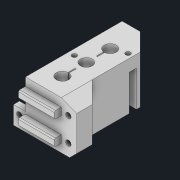
# Autodesk Inventor part: z-bottom
Saved by Autodesk Inventor 2021 (Build 250183000, 183)
## iProperties
Created: 2021-03-14
Part Number: z-bottom
Material: Generic
Document SubType Name: Modeling
Designer: Alex
Density: 1 g/cm^3
Appearance: Default
Author: Alex
## iProperties of the stored document _3DPrint.ipt
Created: 2021-05-20
Part Number: _3DPrint
Material: Generic
Document SubType Name: Modeling
Designer: arbra
Density: 1 g/cm^3
Appearance: Default
Author: arbra
Autodesk Inventor part; units mm, degrees
ref_plane "YZ Plane" through (0, 0, 0) normal (1, 0, 0) x (0, 1, 0)
ref_plane "XZ Plane" through (0, 0, 0) normal (0, 1, 0) x (-1, 0, 0)
sketch "Sketch1" plane through (0, 0, 0) normal (0, 1, 0) x (-1, 0, 0)
  circle A0 centre (0, 0) radius 5
  line L0 (-23.6, 0) -> (36.6, 0) construction
  line L1 (0, -52.2) -> (0, 61.2) construction
  circle A1 centre (0, 20) radius 5.125
  circle A2 centre (0, -20) radius 5.125
  circle A3 centre (-10, 0) radius 2
  circle A4 centre (11, 24) radius 2
  line L2 (0, 45) -> (15, 30)
  line L3 (15, 30) -> (15, -10)
  line L4 (15, -10) -> (28, -23)
  line L5 (28, -23) -> (28, -36)
  line L6 (28, -36) -> (-15, -36)
  line L7 (-15, -36) -> (-15, 45)
  line L8 (-15, 45) -> (0, 45)
  line L9 (0.375, 14.8887) -> (0.375, 8.8887)
  line L10 (0.375, 8.8887) -> (-0.375, 8.8887)
  line L11 (-0.375, 8.8887) -> (-0.375, 14.8887)
  line L12 (0.375, -14.8887) -> (0.375, -8.8887)
  line L13 (0.375, -8.8887) -> (-0.375, -8.8887)
  line L14 (-0.375, -8.8887) -> (-0.375, -14.8887)
  dimension "d0" = 10
  dimension "d1" = 10.25
  dimension "d3" = 40
  dimension "d4" = 4
  dimension "d5" = 11
  dimension "d6" = 4
  dimension "d9" = 10
  dimension "d10" = 4
  dimension "d13" = 45
  dimension "d14" = 15
  dimension "d16" = 16
  dimension "d17" = 13
  dimension "d18" = 45
  dimension "d19" = 25
  dimension "d24" = 0.75
  dimension "d25" = 6
  dimension "d106" = 13
  constraints: 26 end point, 5 centre point, 5 perpendicular, 5 symmetric about line, 4 point on line, 2 equal radius, 2 point on circle, 2 vertical, 1 coincident, 1 parallel, 1 other
  measures "d0" diameter of A0
  measures "d1" diameter of A1
  measures "d3" distance of A2.centre A1.centre
  measures "d4" diameter of A4
  measures "d5" horizontal distance of A4.centre A1.centre
  measures "d6" vertical distance of A4.centre A1.centre
  measures "d9" distance of A3.centre A0.centre
  measures "d10" distance from line of L3 A4.centre
  measures "d13" angle of L3 L4
  measures "d14" distance from line of L7 A0.centre
  measures "d16" distance from line of L6 A2.centre
  measures "d17" distance of L4.end L5.end
  measures "d18" angle of L2 L8
  measures "d19" distance from line of L8 A1.centre
  measures "d24" distance of L9.end L10.end
  measures "d25" distance of L9.start L9.end
  measures "d106" distance between parallel lines of L5 L3
extrude "Extrusion1" add sketch "Sketch1" along normal blind 40
sketch "Sketch2" plane through (0, 0, 0) normal (0, -1, 0) x (1, 0, 0)
  circle A0 centre (0, 0) radius 5 projected
extrude "Extrusion2" add sketch "Sketch2" against normal blind 20
sketch "Sketch3" plane through (0, 0, 0) normal (0, -1, 0) x (1, 0, 0)
  arc A0 (-0.375, -14.8887) -> (0.375, -14.8887) centre (0, -20) ccw projected
  circle A1 centre (0, -20) radius 2.5
  line L0 (-36.6, 0) -> (23.6, 0) construction
  line L1 (0.375, -14.8887) -> (0.375, -8.8887) projected
  line L2 (-0.375, -8.8887) -> (-0.375, -14.8887) projected
  line L3 (0.375, -8.8887) -> (-0.375, -8.8887) projected
  line L4 (-0.375, -14.8887) -> (-0.375, -17.5283)
  line L5 (0.375, -14.8887) -> (0.375, -17.5283)
  line L6 (-0.375, -22.4717) -> (-0.375, -24.9717)
  line L7 (-0.375, -24.9717) -> (0.375, -24.9717)
  line L8 (0.375, -24.9717) -> (0.375, -22.4717)
  arc A2 (0.375, 14.8887) -> (-0.375, 14.8887) centre (0, 20) ccw projected
  line L9 (-0.375, 14.8887) -> (-0.375, 8.8887) projected
  line L10 (0.375, 8.8887) -> (0.375, 14.8887) projected
  line L11 (-0.375, 8.8887) -> (0.375, 8.8887) projected
  circle A3 centre (0, 20) radius 2.5
  line L12 (-0.375, 14.8887) -> (-0.375, 17.5283)
  line L13 (0.375, 14.8887) -> (0.375, 17.5283)
  line L14 (-0.375, 22.4717) -> (-0.375, 24.9717)
  line L15 (-0.375, 24.9717) -> (0.375, 24.9717)
  line L16 (0.375, 24.9717) -> (0.375, 22.4717)
  line L17 (-0.375, -8.8887) -> (-0.375, -14.8887) projected
  arc A4 (0.375, -14.8887) -> (-0.375, -14.8887) centre (0, -20) ccw
  arc A5 (-0.375, 14.8887) -> (0.375, 14.8887) centre (0, 20) ccw
  point P0 (0, 0)
  dimension "d26" = 5
  dimension "d27" = 2.5
  dimension "d30" = 5.125
  dimension "d31" = 5.125
  constraints: 20 end point, 12 point on circle, 8 symmetric about line, 4 centre point, 3 vertical, 2 collinear, 1 coincident, 1 horizontal, 1 perpendicular, 2 other
  measures "d26" diameter of A1
  measures "d27" distance of L6.start L6.end
  measures "d30" radius of A4
  measures "d31" radius of A0
extrude "Extrusion3" add sketch "Sketch3" against normal blind 3.5 contours L4 A1 L6 L7 L8 L5 A0 | L2 L3 L1 A4 | L13 A3 L16 L15 L14 L12 A2 | L10 L11 L9 A5
sketch "Sketch4" plane through (15, 0, 45) normal (1, 0, 0) x (0, 0, -1)
  line L0 (81, 0) -> (81, 40) construction
  line L1 (81, 33.145) -> (85.85, 33.145)
  line L2 (86.85, 32.145) -> (86.85, 27.855)
  line L3 (85.85, 26.855) -> (81, 26.855)
  line L4 (81, 26.855) -> (81, 33.145)
  line L5 (81, 20) -> (108.6331, 20) construction
  line L6 (0, 40) -> (81, 40) construction
  line L7 (85.85, 33.145) -> (86.85, 32.145)
  line L8 (85.85, 26.855) -> (86.85, 27.855)
  line L9 (81, 6.855) -> (85.85, 6.855)
  line L10 (86.85, 7.855) -> (86.85, 12.145)
  line L11 (85.85, 13.145) -> (81, 13.145)
  line L12 (81, 13.145) -> (81, 6.855)
  line L13 (85.85, 6.855) -> (86.85, 7.855)
  line L14 (85.85, 13.145) -> (86.85, 12.145)
  point P0 (45, 0)
  point P1 (86.85, 26.855)
  point P2 (86.85, 33.145)
  point P3 (86.85, 13.145)
  point P4 (86.85, 6.855)
  dimension "d32" = 6.855
  dimension "d33" = 5.85
  dimension "d34" = 6.29
  dimension "d35" = 1
  dimension "d36" = 1
  dimension "d37" = 1
  dimension "d38" = 1
  constraints: 26 end point, 9 point on line, 8 symmetric about line, 2 horizontal, 2 parallel, 1 midpoint, 1 perpendicular
  measures "d32" distance between parallel lines of L1 L6
  measures "d33" distance of L1.start point (86.85, 33.145)
  measures "d34" distance between parallel lines of L3 L1
  measures "d35" distance of L1.end point (86.85, 33.145)
  measures "d36" distance of L2.start point (86.85, 33.145)
  measures "d37" distance of L3.start point (86.85, 26.855)
  measures "d38" distance of L2.end point (86.85, 26.855)
extrude "Extrusion4" add sketch "Sketch4" against normal up to surface (43 mm away)
sketch "Sketch5" plane through (15, 27.855, -41.85) normal (0, 0, -1) x (-1, 0, 0)
  line L0 (30, -27.855) -> (30, 12.145) construction
  line L1 (0, 5.29) -> (43, 5.29) projected
  line L2 (36, 5.29) -> (36, -1) construction
  line L3 (43, -1) -> (0, -1) projected
  circle A0 centre (36, 2.145) radius 2.25
  line L4 (0, -27.855) -> (0, 12.145) projected
  line L5 (0, -7.855) -> (43, -7.855) construction
  line L6 (43, -27.855) -> (43, 12.145) projected
  circle A1 centre (36, -17.855) radius 2.25
  point P0 (15, -27.855)
  dimension "d41" = 4.5
  dimension "d42" = 6
  constraints: 4 end point, 3 midpoint, 2 centre point, 2 point on line, 1 symmetric about line, 1 vertical, 1 other
  measures "d41" diameter of A0
  measures "d42" distance from line of L0 A0.centre
extrude "Extrusion5" cut sketch "Sketch5" against normal through all contours A0 | A1
ref_plane "Work Plane1" through (-15, 0, -10) normal (0, 0, 1) x (0, 1, 0)
sketch "Sketch6" plane through (-15, 0, -10) normal (0, 0, 1) x (0, 1, 0)
  circle A0 centre (30, 6) radius 2.25 projected
  circle A1 centre (30, 6) radius 3.75
  circle A2 centre (10, 6) radius 2.25 projected
  circle A3 centre (10, 6) radius 3.75
  point P0 (0, -15)
  dimension "d46" = 7.5
  dimension "d47" = 7.5
  constraints: 2 centre point, 2 coincident
  measures "d46" diameter of A1
  measures "d47" diameter of A3
extrude "Extrusion6" cut sketch "Sketch6" against normal blind 21 contours A0 | A1 | A2 | A3
sketch "Sketch7" plane through (15, 27.855, -41.85) normal (0, 0, -1) x (-1, 0, 0)
  line L0 (0, -27.855) -> (0, 12.145) projected
  line L1 (0, -7.855) -> (43, -7.855) construction
  line L2 (43, -27.855) -> (43, 12.145) projected
  line L3 (0, -15.71) -> (0, -20)
  line L4 (0, -12.855) -> (-10, -12.855)
  line L5 (-10, -12.855) -> (-10, -27.855)
  line L6 (-10, -27.855) -> (0, -27.855)
  line L7 (0, -27.855) -> (0, -12.855)
  line L8 (15, -27.855) -> (0, -27.855) projected
  point P0 (0, 0)
  point P1 (0, 4.29)
  point P2 (0, -17.855)
  point P3 (0, -12.855)
  point P4 (-10, -20.355)
  dimension "d63" = 10
  dimension "d64" = 5
  constraints: 12 end point, 3 midpoint, 2 collinear, 2 symmetric about line, 1 horizontal, 1 vertical
  measures "d63" distance of L4.start L5.start
  measures "d64" distance between parallel lines of L4 L1
extrude "Extrusion7" add sketch "Sketch7" against normal up to surface (86.85 mm away)
sketch "Sketch9" plane through (-28, 27.855, -41.85) normal (0, 0, -1) x (-1, 0, 0)
  arc A0 (-6.3207, 0) -> (-6.3207, 4.29) centre (-7, 2.145) ccw projected
  line L0 (-43, -6.9275) -> (0, -7.855) construction
  line L1 (0, -14.71) -> (0, -1) projected
  circle A1 centre (-48, -17.855) radius 2.25
  line L2 (-43, -12.855) -> (-53, -12.855) projected
  arc A2 (-7.6793, -15.71) -> (-7.6793, -20) centre (-7, -17.855) ccw projected
  line L3 (-7, -17.855) -> (-48, -17.855) construction
  line L4 (-48, -12.855) -> (-48, -17.855) construction
  point P0 (-28, -27.855)
  constraints: 6 end point, 2 midpoint, 1 centre point, 1 equal radius, 1 horizontal, 1 vertical
extrude "Extrusion9" cut sketch "Sketch9" against normal through all
sketch "Sketch10" plane through (0, 0, 45) normal (0, 0, 1) x (1, 0, 0)
  circle A0 centre (20, 10) radius 2.25 projected
  circle A1 centre (20, 10) radius 3.5
  point P0 (0, 0)
  dimension "d59" = 7
  constraints: 1 centre point, 1 coincident
  measures "d59" diameter of A1
extrude "Extrusion10" cut sketch "Sketch10" against normal blind 70 contours A0 | A1
sketch "Sketch11" plane through (25, 0, -41.85) normal (1, 0, 0) x (0, 0, -1)
  line L0 (-1, 13.145) -> (-5.85, 13.145) projected
  line L1 (-5.85, 13.145) -> (-5.85, 15) projected
  line L2 (0, 15) -> (-5.85, 15) projected
  line L3 (0, 12.145) -> (0, 15) projected
  line L4 (0, 12.145) -> (-1, 13.145) projected
  line L5 (-5.85, 13.145) -> (-5.85, 6.855) projected
  line L6 (0, 0) -> (0, 7.855) projected
  line L7 (-1, 6.855) -> (0, 7.855) projected
  line L8 (-5.85, 6.855) -> (-1, 6.855) projected
  line L9 (-5.85, 0) -> (-5.85, 6.855) projected
  line L10 (-5.85, 6.855) -> (-5.85, 0)
  line L11 (0, 0) -> (-86.85, 0) projected
  line L12 (-5.85, 0) -> (0, 0)
  point P0 (-41.85, 0)
  constraints: 4 end point, 1 collinear, 1 vertical
extrude "Extrusion11" cut sketch "Sketch11" against normal through all
sketch "Sketch12" plane through (15, 27.855, -41.85) normal (1, 0, 0) x (0, 0, -1)
  line L0 (-43.85, 12.145) -> (-39.85, 12.145) projected
  line L1 (-44.85, -27.855) -> (-38.85, -27.855)
  line L2 (-38.85, -27.855) -> (-38.85, 2.145)
  line L3 (-38.85, 2.145) -> (-44.85, 2.145)
  line L4 (-44.85, 2.145) -> (-44.85, -27.855)
  line L5 (-41.85, 12.145) -> (-41.85, 2.145)
  line L6 (-31.85, -27.855) -> (-71.85, -27.855) projected
  point P0 (-41.85, -27.855)
  dimension "d72" = 10
  dimension "d74" = 6
  constraints: 10 end point, 2 midpoint, 2 parallel, 2 perpendicular, 1 collinear, 1 horizontal, 1 other
  measures "d72" distance between parallel lines of L3 L0
  measures "d74" distance of L1.start L1.end
extrude "Extrusion12" cut sketch "Sketch12" against normal blind 8
sketch "Sketch13" plane through (-15, 10, -10) normal (-1, 0, 0) x (0, 0, 1)
  line L0 (32, 30) -> (36, 30) projected
  line L1 (34, 30) -> (34, 20)
  line L2 (31, -10) -> (37, -10)
  line L3 (37, -10) -> (37, 20)
  line L4 (37, 20) -> (31, 20)
  line L5 (31, 20) -> (31, -10)
  line L6 (0, -10) -> (40, -10) projected
  dimension "d79" = 6
  dimension "d110" = 10
  constraints: 10 end point, 2 midpoint, 2 parallel, 1 collinear, 1 horizontal, 1 perpendicular, 1 other
  measures "d79" distance of L2.start L2.end
  measures "d110" distance between parallel lines of L4 L0
extrude "Extrusion13" cut sketch "Sketch13" against normal blind 8
chamfer "Chamfer2" distance 13 distance2 5 1 edges at (-28, 40, -29.5) measured on face at (-4.5425, 40, -32.3621)
chamfer "Chamfer3" distance 6 angle 45 1 edges at (-28, 0, -29.5)
sketch "Sketch18" plane through (15, 15, -36) normal (0, 1, 0) x (1, 0, 0)
  line L0 (-37, -19) -> (-43, -13) construction
  line L1 (10, 0) -> (10, -81) projected
  line L2 (0, -81) -> (0, 0) projected
  line L3 (10, 0) -> (0, 0)
  line L4 (0, 0) -> (0, -5)
  line L5 (0, -5) -> (10, -5)
  line L6 (10, -5) -> (10, 0)
  line L7 (10, 0) -> (10, -81) projected
  line L8 (10, -81) -> (0, -81)
  line L9 (8.5, -81) -> (1.5, -81) projected
  point P0 (-15, -36)
  point P1 (10, -5)
  dimension "d109" = 5
  constraints: 10 end point, 2 parallel, 1 collinear, 1 horizontal, 1 perpendicular, 1 point on line
  measures "d109" distance between parallel lines of L3 L5
extrude "Extrusion18" cut sketch "Sketch18" against normal through all contours L1 L8 L2 L5
sketch "Sketch20" plane through (0, 40, 0) normal (0, 1, 0) x (1, 0, 0)
  line L0 (17.75, 41.85) -> (22.25, 41.85) projected
  line L1 (-20.3207, 41.85) -> (-18.75, 41.85) projected
  line L2 (25, 36) -> (15, 36)
  line L3 (15, 36) -> (15, 41.85)
  line L4 (15, 41.85) -> (25, 41.85)
  line L5 (25, 41.85) -> (25, 36)
  line L6 (25, 40.85) -> (25, 36) projected
  line L7 (25, 36) -> (15, 36) projected
  line L8 (25, 41.85) -> (-28, 41.85) construction
  line L9 (15, 40.85) -> (15, 36) projected
  line L10 (-28, 41.85) -> (-15, 41.85)
  line L11 (-15, 41.85) -> (-15, 36)
  line L12 (-15, 36) -> (-28, 36)
  line L13 (-28, 36) -> (-28, 41.85)
  line L14 (-15, 36) -> (-28, 36) projected
  line L15 (-28, 40.85) -> (-28, 36) projected
  line L16 (15, 41.85) -> (-28, 41.85) construction
  line L17 (-15, 10) -> (-15, 36) projected
  point P0 (0, 0)
  constraints: 16 end point, 8 collinear, 4 parallel, 2 horizontal, 2 perpendicular
extrude "Extrusion19" cut sketch "Sketch20" against normal through all
equation "\"d30\" = d31"
equation "\"d36\" = d35"
equation "\"d37\" = d35"
equation "\"d38\" = d37"
equation "\"d47\" = d46"
equation "\"d79\" = d74"
body "Solid1"
